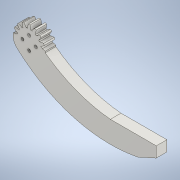
# Autodesk Inventor part: Spur Gear1
Saved by Autodesk Inventor 2020 (Build 240168000, 168)
## iProperties
CustomPartVersion: 1
Created: 2020-01-21
Part Number: Spur Gear1
Material: Steel
Document SubType Name: Modeling
Designer: piolo.pulanco
Categories: <?xml version="1.0" encoding="UTF-16"?> <MemberInstance><Categories><FamilyTemplate><FamilyTemplateParameter ValueType="xs:double" Id="1" ObjectReferenceKey="da_z" ObjectType="kUserParameterObject"/><FamilyTemplateParameter ValueType="xs:double" Id="2" ObjectReferenceKey="da_b" ObjectType="kUserParameterObject"/><FamilyTemplateParameter ValueType="xs:double" Id="3" ObjectReferenceKey="da_beta" ObjectType="kUserParameterObject"/><FamilyTemplateParameter ValueType="xs:double" Id="4" ObjectReferenceKey="da_da" ObjectType="kUserParameterObject"/><FamilyTemplateParameter ValueType="xs:double" Id="5" ObjectReferenceKey="da_aw" ObjectType="kUserParameterObject"/><FamilyTemplateParameter ValueType="xs:string" Id="6" ObjectReferenceKey="EAIAABAAAAC/AAAAAAAAAIAAAAAAAAAA" ObjectType="83910656" SubObjectId="SurfaceGeometry"/></FamilyTemplate><ParamToTemplateMap><ParamToTemplate CategoryParameter="//CategoryParameter[@InternalName='046C89C9-8512-4d59-83FE-43B91F4F132A']" TemplateParameter="1"/><ParamToTemplate CategoryParameter="//CategoryParameter[@InternalName='2552DF32-E462-4b46-AEBF-C6C7768E72AC']" TemplateParameter="2"/><ParamToTemplate CategoryParameter="//CategoryParameter[@InternalName='C9EE641D-15FC-4fae-A226-E94C4372FDD7']" TemplateParameter="3"/><ParamToTemplate><ParamToTemplate CategoryParameter="//CategoryParameter[@InternalName='00B6519A-459B-49c7-AD84-2E56D39A5744']" ConstantValue="0.050708"/></ParamToTemplate><ParamToTemplate><ParamToTemplate CategoryParameter="//CategoryParameter[@InternalName='04B31F0E-C7A6-4894-AA32-9629BEFACF47']" ConstantValue="1.000000"/></ParamToTemplate><ParamToTemplate><ParamToTemplate CategoryParameter="//CategoryParameter[@InternalName='43CBEC2E-7847-49e7-A936-2F7889FCB2D9']" ConstantValue="0.250000"/></ParamToTemplate><ParamToTemplate><ParamToTemplate CategoryParameter="//CategoryParameter[@InternalName='B1EFC894-105D-4ebd-86BF-FA20ED196853']" ConstantValue="0.333500"/></ParamToTemplate><ParamToTemplate><ParamToTemplate CategoryParameter="//CategoryParameter[@InternalName='51175063-3D10-4879-93E8-6246FE8B403D']" ConstantValue="2061532430.657340"/></ParamToTemplate><ParamToTemplate><ParamToTemplate CategoryParameter="//CategoryParameter[@InternalName='A3A52E27-4454-46a9-B0BD-C932399B70AF']" ConstantValue="0.300000"/></ParamToTemplate><ParamToTemplate><ParamToTemplate CategoryParameter="//CategoryParameter[@InternalName='91B76062-C214-41d9-B1B9-14D2AB99603D']" ConstantValue="0.211667"/></ParamToTemplate><ParamToTemplate><ParamToTemplate CategoryParameter="//CategoryParameter[@InternalName='374E806E-8B8A-4dda-A9AA-1039D6500AD2']" ConstantValue="4.724409"/></ParamToTemplate><ParamToTemplate><ParamToTemplate CategoryParameter="//CategoryParameter[@InternalName='2D373A89-B862-43d6-8D0B-0CBF12AB9F6C']" ConstantValue="0.349066"/></ParamToTemplate><ParamToTemplate CategoryParameter="//CategoryParameter[@InternalName='37777632-D6A2-4fac-9D53-DB8ACD95C989']" TemplateParameter="4"/><ParamToTemplate CategoryParameter="//CategoryParameter[@InternalName='FD1017F1-B727-4f7e-9707-0F86F1FF9423']" TemplateParameter="5"/><ParamToTemplate><ParamToTemplate CategoryParameter="//CategoryParameter[@InternalName='9E1B4470-B2D3-4ff1-B813-535BB4CDF51A']" ConstantValue="3523220.976809"/></ParamToTemplate><ParamToTemplate><ParamToTemplate CategoryParameter="//CategoryParameter[@InternalName='F8452263-BFF6-458c-9FB1-07C4B99E95CD']" ConstantValue="11397033.805607"/></ParamToTemplate><ParamToTemplate><ParamToTemplate CategoryParameter="//CategoryParameter[@InternalName='3E3BB259-FD49-497f-8171-6EBC954A3479']" ConstantValue="2.000000"/></ParamToTemplate><ParamToTemplate CategoryParameter="//CategoryParameter[@InternalName='27C3BAF2-7550-4e4b-AE2C-0DB134B7D9B7']" TemplateParameter="6"/></ParamToTemplateMap><Category DisplayName="Gear" InternalName="DC85795E-93AB-48d5-8EEE-5A27447B64BD" Mnemonic="Gear"><CategoryParameter DisplayName="z" InternalName="046C89C9-8512-4d59-83FE-43B91F4F132A" Mnemonic="z"/><CategoryParameter DisplayName="b" InternalName="2552DF32-E462-4b46-AEBF-C6C7768E72AC" Mnemonic="b"/><CategoryParameter DisplayName="||b|" InternalName="C9EE641D-15FC-4fae-A226-E94C4372FDD7" Mnemonic="beta"/><CategoryParameter DisplayName="x" InternalName="00B6519A-459B-49c7-AD84-2E56D39A5744" Mnemonic="x"/><CategoryParameter DisplayName="a*" InternalName="04B31F0E-C7A6-4894-AA32-9629BEFACF47" Mnemonic="a"/><CategoryParameter DisplayName="c*" InternalName="43CBEC2E-7847-49e7-A936-2F7889FCB2D9" Mnemonic="c"/><CategoryParameter DisplayName="r|.f|*" InternalName="B1EFC894-105D-4ebd-86BF-FA20ED196853" Mnemonic="rf"/><CategoryParameter DisplayName="E" InternalName="51175063-3D10-4879-93E8-6246FE8B403D" Mnemonic="E"/><CategoryParameter DisplayName="||m|" InternalName="A3A52E27-4454-46a9-B0BD-C932399B70AF" Mnemonic="mi"/><Category DisplayName="SpurGear" InternalName="26C5A22E-A91E-4dfd-A3B3-23CCAFAE1764" Mnemonic="SpurGear"><CategoryParameter DisplayName="m" InternalName="91B76062-C214-41d9-B1B9-14D2AB99603D" Mnemonic="m"/><CategoryParameter DisplayName="P" InternalName="374E806E-8B8A-4dda-A9AA-1039D6500AD2" Mnemonic="PP"/><CategoryParameter DisplayName="||a|" InternalName="2D373A89-B862-43d6-8D0B-0CBF12AB9F6C" Mnemonic="alpha"/><CategoryParameter DisplayName="d|.a|" InternalName="37777632-D6A2-4fac-9D53-DB8ACD95C989" Mnemonic="da"/><CategoryParameter DisplayName="a|.w|" InternalName="FD1017F1-B727-4f7e-9707-0F86F1FF9423" Mnemonic="aw"/><CategoryParameter DisplayName="||s||.Flim|" InternalName="9E1B4470-B2D3-4ff1-B813-535BB4CDF51A" Mnemonic="sFlim"/><CategoryParameter DisplayName="||s||.Hlim|" InternalName="F8452263-BFF6-458c-9FB1-07C4B99E95CD" Mnemonic="sHlim"/><CategoryParameter DisplayName="type" InternalName="3E3BB259-FD49-497f-8171-6EBC954A3479" Mnemonic="type"/><CategoryParameter DisplayName="PitchDiameter" InternalName="27C3BAF2-7550-4e4b-AE2C-0DB134B7D9B7" Mnemonic="IDS_PITCHDIAM"/></Category></Category></Categories></MemberInstance>
Density: 1 g/cm^3
Appearance: Steel
d9: 0.000 in
d14: 0.000 in
d15: 1.342 in
d16: 0.000 in
d17: 0.000 in
d18: 0.000 in
d19: 1.342 in
Author: piolo.pulanco
Autodesk Inventor part; units mm, degrees
ref_plane "YZ Plane" through (0, 0, 0) normal (1, 0, 0) x (0, 1, 0)
ref_plane "XZ Plane" through (0, 0, 0) normal (0, 1, 0) x (-1, 0, 0)
ref_plane "XY Plane" through (0, 0, 0) normal (0, 0, 1) x (1, 0, 0)
sketch "Sketch1" plane through (0, 0, 0) normal (0, 0, 1) x (1, 0, 0)
  circle A0 centre (0, 0) radius 19.1525
  dimension "d0" = 38.3051
  constraints: 1 centre point
  measures "d0" diameter of A0
extrude "Extrusion1" add sketch "Sketch1" along normal blind 12.7
sketch "Sketch2" plane through (0, 0, 0) normal (0, 0, -1) x (-1, 0, 0)
  circle A0 centre (0, 0) radius 19.1525 projected
  circle A1 centre (0, 0) radius 17.0383
  dimension "d3" = 34.0766
  constraints: 1 centre point, 1 coincident
  measures "d3" diameter of A1
surface extrude "Pitch Diameter" sketch "Sketch2" against normal through all shown no curves A1
ref_plane "Work Plane1" through (0, 0, 0) normal (1, 0, 0) x (0, 1, 0)
ref_plane "Work Plane2" through (0, 0, 0) normal (0.9807853, 0.1950903, 0) x (0, 0, 1)
ref_plane "Work Plane3" through (0, 0, 6.35) normal (0, 0, -1) x (-1, 0, 0)
spur gear teeth "Spur Gear" teeth 16 pitch diameter 33.8667 tip diameter 38.305 root diameter 28.7897 face width 12.7 start plane through (0, 0, 0) normal (0, 0, -1) x (-1, 0, 0)
sketch "Sketch3" plane through (0, 0, 12.7) normal (0, 0, 1) x (1, 0, 0)
  circle A0 centre (0, 0) radius 8.001
  circle A1 centre (0, 8.001) radius 1.7907
  circle A2 centre (8.001, 0) radius 1.7907
  circle A3 centre (-8.001, 0) radius 1.7907
  circle A4 centre (0, -8.001) radius 1.7907
  dimension "d67" = 16.002
  dimension "d68" = 3.5814
  dimension "d69" = 3.5814
  dimension "d70" = 3.5814
  dimension "d71" = 3.5814
  constraints: 5 centre point, 4 point on circle, 1 coincident
  measures "d67" diameter of A0
  measures "d68" diameter of A1
  measures "d69" diameter of A2
  measures "d70" diameter of A3
  measures "d71" diameter of A4
extrude "Extrusion2" cut sketch "Sketch3" against normal blind 25.4 contours A0 A2 | A0 A2 | A1 A0 | A0 A1 | A4 A0 | A0 A4 | A3 A0 | A0 A3
sketch "Sketch4" plane through (0, 0, 12.7) normal (0, 0, 1) x (1, 0, 0)
  line L0 (0, 0) -> (0, -31.6611)
  line L1 (0, -31.6611) -> (127, -31.6611)
  line L2 (127, -31.6611) -> (127, -72.7724)
  arc A0 (0, 0) -> (127, -42.2564) centre (111.8867, 124.2962) ccw construction
  arc A1 (-2.7161, -13.0272) -> (128.0505, -53.8337) centre (111.8867, 124.2962) ccw
  arc A2 (13.7906, 3.4977) -> (125.9495, -30.6792) centre (111.8867, 124.2962) ccw
  arc A3 (128.0505, -53.8337) -> (125.9495, -30.6792) centre (127, -42.2564) ccw
  arc A4 (-2.7161, -13.0272) -> (13.7906, 3.4977) centre (-4.9514, 5.7124) ccw
  point P0 (0, 11.6248)
  dimension "d27" = 31.6611
  dimension "d28" = 127
  constraints: 10 point on circle, 6 end point, 5 centre point, 2 point on line, 2 tangent, 2 vertical, 1 perpendicular
  measures "d27" distance of L0.start L0.end
  measures "d28" distance of L0.end L1.end
extrude "Extrusion3" add sketch "Sketch4" against normal blind 12.7 contours A4 A2 A3 A1 L2 L1 L0 | L0 A1 A4 | L1 L2 A1
sketch "Sketch6" plane through (0, 0, 12.7) normal (0, 0, 1) x (1, 0, 0)
  arc A0 (-12.7151, -6.4873) -> (119.3661, -46.968) centre (99.5244, 124.0111) ccw construction
  arc A1 (-16.1505, -10.4816) -> (119.9734, -52.2013) centre (99.5244, 124.0111) ccw
  arc A2 (-9.2797, -2.493) -> (118.7588, -41.7347) centre (99.5244, 124.0111) ccw
  arc A3 (-9.2797, -2.493) -> (-16.1505, -10.4816) centre (-12.7151, -6.4873) ccw
  arc A4 (119.9734, -52.2013) -> (118.7588, -41.7347) centre (119.3661, -46.968) ccw
  point P0 (0, 0)
  constraints: 10 point on circle, 5 centre point, 4 tangent
extrude "Extrusion4" add sketch "Sketch6" against normal blind 12.7
sketch "Sketch7" plane through (0, 0, 12.7) normal (0, 0, 1) x (1, 0, 0)
  arc A0 (128.0505, -53.8337) -> (125.9495, -30.6792) centre (127, -42.2564) ccw projected
  line L0 (127, -30.6316) -> (88.9, -30.6316)
  line L1 (88.9, -30.6316) -> (88.9, -43.3316)
  line L2 (88.9, -43.3316) -> (127, -43.3316)
  line L3 (127, -43.3316) -> (127, -30.6316)
  line L4 (127, -43.3316) -> (152.4, -43.3316)
  line L5 (152.4, -43.3316) -> (152.4, -30.6316)
  line L6 (152.4, -30.6316) -> (127, -30.6316)
  line L7 (127, -30.6316) -> (127, -43.3316)
  point P0 (0, 0)
  dimension "d33" = 38.1
  dimension "d34" = 12.7
  dimension "d35" = 25.4
  constraints: 16 end point, 4 parallel, 2 horizontal, 2 perpendicular, 1 point on circle, 1 point on line
  measures "d33" distance of L2.end L1.end
  measures "d34" distance of L1.end L0.end
  measures "d35" distance of L6.end L5.end
extrude "Extrusion5" add sketch "Sketch7" against normal blind 12.7
sketch "Sketch8" plane through (0, 0, 12.7) normal (0, 0, 1) x (1, 0, 0)
  arc A0 (-13.7822, -8.8488) -> (39.9833, -39.4768) centre (70.5618, 76.7068) ccw construction
  arc A1 (-16.0548, -11.1541) -> (39.1593, -42.6073) centre (70.5618, 76.7068) ccw
  arc A2 (-11.5096, -6.5435) -> (40.8072, -36.3463) centre (70.5618, 76.7068) ccw
  arc A3 (-11.5096, -6.5435) -> (-16.0548, -11.1541) centre (-13.7822, -8.8488) ccw
  arc A4 (39.1593, -42.6073) -> (40.8072, -36.3463) centre (39.9833, -39.4768) ccw
  point P0 (0, 0)
  constraints: 10 point on circle, 5 centre point, 4 tangent
extrude "Extrusion6" add sketch "Sketch8" against normal blind 12.7
sketch "Sketch9" plane through (0, 0, 12.7) normal (0, 0, 1) x (1, 0, 0)
  line L0 (152.4, -43.3316) -> (138.575, -43.3316) projected
  arc A0 (128.0505, -53.8337) -> (138.575, -43.3316) centre (127, -42.2564) ccw projected
  line L1 (152.4, -43.3316) -> (131.8736, -52.8103)
  line L2 (131.8736, -52.8103) -> (129.0618, -46.7213)
  line L3 (129.0618, -46.7213) -> (149.5882, -37.2426)
  line L4 (149.5882, -37.2426) -> (152.4, -43.3316)
  point P0 (0, 0)
  constraints: 8 end point, 2 parallel, 1 perpendicular, 1 point on circle, 1 tangent
extrude "Extrusion7" add sketch "Sketch9" against normal blind 12.7 contours L1 A0 L0
sketch "Sketch11" plane through (0, 0, 12.7) normal (0, 0, 1) x (1, 0, 0)
  arc A0 (-19.1295, -0.9398) -> (-15.4393, -1.9779) centre (-13.1155, 13.3604) ccw projected
  arc A1 (-17.9825, -6.5917) -> (-16.9134, -9.6702) centre (-12.7151, -6.4873) ccw projected
  line L0 (-19.1295, -0.9398) -> (-17.7327, -8.0934)
  line L1 (-17.7327, -8.0934) -> (-14.2646, -7.4162)
  line L2 (-14.2646, -7.4162) -> (-15.6613, -0.2626)
  line L3 (-15.6613, -0.2626) -> (-19.1295, -0.9398)
  point P0 (0, 0)
  constraints: 8 end point, 2 parallel, 1 perpendicular, 1 point on circle
extrude "Extrusion9" add sketch "Sketch11" against normal blind 12.7 contours L0 L3 L2 L1
sketch "Sketch12" plane through (0, 0, 12.7) normal (0, 0, 1) x (1, 0, 0)
  arc A0 (-17.9684, -6.8866) -> (-16.9134, -9.6702) centre (-12.7151, -6.4873) ccw projected
  arc A1 (-16.9134, -9.6702) -> (-16.0548, -11.1541) centre (-13.7822, -8.8488) ccw projected
  arc A2 (-17.6717, -8.2728) -> (-16.0719, -11.137) centre (-10.7329, -6.2761) ccw
  line L0 (-17.6717, -8.2728) -> (-15.4773, -9.1763)
  line L1 (-15.4773, -9.1763) -> (-16.0719, -11.137)
  point P0 (0, 0)
  constraints: 4 end point, 4 point on circle, 1 centre point
extrude "Extrusion10" add sketch "Sketch12" against normal blind 12.7 contours L0 L1 A2 A1 A0 | A0 A1 A2
sketch "Sketch13" plane through (0, 0, 12.7) normal (0, 0, 1) x (1, 0, 0)
  arc A0 (-12.862, -14.1911) -> (37.1919, -42.0721) centre (70.5618, 76.7068) ccw projected
  arc A1 (-19.1453, 0.8258) -> (-16.0548, -11.1541) centre (-3.912, -1.633) ccw
  line L0 (-19.1453, 0.8258) -> (-16.0548, -11.1541)
  point P0 (0, 0)
  point P1 (-13.0703, -13.9996)
  constraints: 2 end point, 2 point on circle, 1 centre point
extrude "Extrusion11" add sketch "Sketch13" against normal blind 12.7
sketch "Sketch15" plane through (0, 0, 12.7) normal (0, 0, 1) x (1, 0, 0)
  arc A0 (-12.862, -14.1911) -> (37.1919, -42.0721) centre (70.5618, 76.7068) ccw projected
  arc A1 (88.6571, -53.0506) -> (128.0505, -53.8337) centre (111.8867, 124.2962) ccw projected
  arc A2 (5.2755, -27.9816) -> (88.6571, -53.0506) centre (98.0913, 129.5298) ccw
  line L0 (5.2755, -27.9816) -> (77.0502, -39.7701)
  line L1 (77.0502, -39.7701) -> (88.6571, -53.0506)
  point P0 (0, 0)
  constraints: 4 end point, 4 point on circle, 1 centre point
extrude "Extrusion13" add sketch "Sketch15" against normal blind 12.7 contours L0 L1 A2
sketch "Sketch17" plane through (0, 0, 12.7) normal (0, 0, 1) x (1, 0, 0)
  arc A0 (-16.0548, -11.1541) -> (-13.0703, -13.9996) centre (70.5618, 76.7068) ccw projected
  arc A1 (128.0505, -53.8337) -> (131.8736, -52.8103) centre (127, -42.2564) ccw projected
  arc A2 (-16.0548, -11.1541) -> (128.0505, -53.8337) centre (97.4568, 107.4898) ccw
  line L0 (-16.0548, -11.1541) -> (131.8736, -52.8103)
  point P0 (0, 0)
  constraints: 2 end point, 2 point on circle, 1 centre point
extrude "Extrusion15" add sketch "Sketch17" against normal blind 12.7
equation "\"d0\" = da_da"
equation "\"d1\" = da_b"
equation "\"d3\" = da_dw"
equation "\"d15\" = da_aw"
equation "\"d19\" = da_aw"
equation "\"da_da\" = 38.305046"
equation "\"da_b\" = 12.7"
equation "\"da_dw\" = 34.076615"
equation "\"da_aw\" = 34.076615"
body "Solid1"
body "Srf1"
